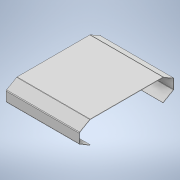
# Autodesk Inventor part: topBody
Saved by Autodesk Inventor 2020.3 (Build 243373000, 373)
## iProperties
Created: 2022-07-13
Part Number: topBody
Material: Generic
Document SubType Name: Sheet Metal
Designer: 0x6f736f646f
Density: 1 g/cm^3
Sheet Metal Rule: Default_mm
Appearance: Default
Author: 0x6f736f646f
Autodesk Inventor part; units mm, degrees
ref_plane "YZ Plane" through (0, 0, 0) normal (1, 0, 0) x (0, 1, 0)
ref_plane "XZ Plane" through (0, 0, 0) normal (0, 1, 0) x (-1, 0, 0)
ref_plane "XY Plane" through (0, 0, 0) normal (0, 0, 1) x (1, 0, 0)
sketch "Sketch1" plane through (0, 0, 0) normal (0, 1, 0) x (-1, 0, 0)
  line L0 (150, 290) -> (-150, 290)
  line L1 (-150, 290) -> (-150, -290)
  line L2 (-150, -290) -> (150, -290)
  line L3 (150, -290) -> (150, 290)
  line L4 (0, -406) -> (0, 406) projected
  line L5 (210, 0) -> (-210, 0) projected
  line L6 (150, 240) -> (-150, 240)
  line L7 (150, 200) -> (-150, 200)
  line L8 (150, 0) -> (-150, 0)
  line L9 (150, -240) -> (-150, -240)
  line L10 (150, -200) -> (-150, -200)
  line L11 (150, 290) -> (110, 240)
  line L12 (110, 200) -> (150, 150)
  line L13 (110, 200) -> (110, 240)
  line L14 (150, -290) -> (110, -240)
  line L15 (110, -200) -> (150, -150)
  line L16 (110, -200) -> (110, -240)
  line L17 (-150, 290) -> (-110, 240)
  line L18 (-110, 200) -> (-150, 150)
  line L19 (-110, 200) -> (-110, 240)
  line L20 (-150, -290) -> (-110, -240)
  line L21 (-110, -200) -> (-150, -150)
  line L22 (-110, -200) -> (-110, -240)
  line L23 (150, 150) -> (-150, 150)
  line L24 (150, -150) -> (-150, -150)
  point P0 (0, 0)
  point P1 (0, -290)
  dimension "d0" = 300
  dimension "d1" = 50
  dimension "d3" = 40
  dimension "d50" = 40
  dimension "d51" = 300
  dimension "d52" = 50
  constraints: 46 end point, 14 symmetric about line, 10 point on line, 3 midpoint, 3 parallel, 2 perpendicular, 1 horizontal, 1 vertical
  measures "d0" distance between parallel lines of L1 L3
  measures "d1" distance between parallel lines of L0 L6
  measures "d3" distance between parallel lines of L6 L7
  measures "d50" distance between parallel lines of L13 L3
  measures "d51" distance between parallel lines of L24 L23
  measures "d52" distance between parallel lines of L23 L7
extrude "Plate1" add sketch "Sketch1" along normal blind 2
fold "Fold7" angle 60 bend radius 2 thickness 2 k factor 0.44 line from (-150, 0, 240) to (150, 0, 240) line at bend centre moving side (0, 0, 1) folds toward (0, -1, 0)
fold "Fold8" angle 60 bend radius 2 thickness 2 k factor 0.44 line from (-150, 0, 200) to (150, 0, 200) line at bend centre moving side (0, 0, 1) folds toward (0, -1, 0)
fold "Fold9" angle 30 bend radius 2 thickness 2 k factor 0.44 line from (-150, 0, 150) to (150, 0, 150) line at bend centre moving side (0, 0, 1) folds toward (0, -1, 0)
fold "Fold10" angle 60 bend radius 2 thickness 2 k factor 0.44 line from (-150, 0, -240) to (150, 0, -240) line at bend centre moving side (0, 0, -1) folds toward (0, -1, 0)
fold "Fold11" angle 60 bend radius 2 thickness 2 k factor 0.44 line from (-150, 0, -200) to (150, 0, -200) line at bend centre moving side (0, 0, -1) folds toward (0, -1, 0)
fold "Fold12" angle 30 bend radius 2 thickness 2 k factor 0.44 line from (-150, 0, -150) to (150, 0, -150) line at bend centre moving side (0, 0, -1) folds toward (0, -1, 0)
equation "\"d5\" = Thickness"
equation "\"d53\" = BendReliefWidth"
equation "\"d54\" = BendReliefDepth"
equation "\"d55\" = MinimumRemnant"
equation "\"d56\" = TransitionRadius"
equation "\"d58\" = BendRadius"
equation "\"d59\" = BendReliefWidth"
equation "\"d60\" = BendReliefDepth"
equation "\"d61\" = MinimumRemnant"
equation "\"d62\" = TransitionRadius"
equation "\"d64\" = BendRadius"
equation "\"d65\" = BendReliefWidth"
equation "\"d66\" = BendReliefDepth"
equation "\"d67\" = MinimumRemnant"
equation "\"d68\" = TransitionRadius"
equation "\"d70\" = BendRadius"
equation "\"d71\" = BendReliefWidth"
equation "\"d72\" = BendReliefDepth"
equation "\"d73\" = MinimumRemnant"
equation "\"d74\" = TransitionRadius"
equation "\"d76\" = BendRadius"
equation "\"d77\" = BendReliefWidth"
equation "\"d78\" = BendReliefDepth"
equation "\"d79\" = MinimumRemnant"
equation "\"d80\" = TransitionRadius"
equation "\"d82\" = BendRadius"
equation "\"d83\" = BendReliefWidth"
equation "\"d84\" = BendReliefDepth"
equation "\"d85\" = MinimumRemnant"
equation "\"d86\" = TransitionRadius"
equation "\"d88\" = BendRadius"
equation "\"BendRadius\" = Thickness"
equation "\"BendReliefWidth\" = Thickness"
equation "\"BendReliefDepth\" = 0.5 * Thickness"
equation "\"CornerReliefSize\" = 4 * Thickness"
equation "\"MinimumRemnant\" = 2 * Thickness"
equation "\"TransitionRadius\" = BendRadius"
equation "\"JacobiRadiusSize\" = BendRadius"
equation "\"GapSize\" = Thickness"
equation "\"Thickness\" = 2"
body "Solid1"
